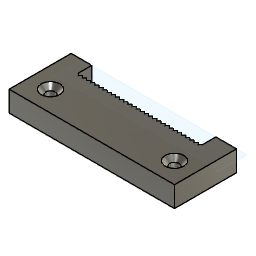
wall holder (Autodesk Fusion 360 design; units mm, degrees)
Autodesk Fusion 360 part; units mm, degrees
note: some values were not read from the file. Chosen so that the rebuilt part matches the saved one: which face or edge a step refers to.
sketch "Skizze1" plane through (0, 0, 0) normal (0, 0, 1) x (1, 0, 0)
  line L0 (0, 0) -> (80, 0)
  line L1 (80, 0) -> (80, -25)
  line L2 (80, -25) -> (0, -25)
  line L3 (0, -25) -> (0, 0)
  line L4 (40, -15) -> (40, -14)
  line L5 (40, -14) -> (39, -15)
  line L6 (38, -14) -> (39, -15)
  line L7 (38, -14) -> (37, -15)
  line L8 (37, -15) -> (36, -14)
  line L9 (36, -14) -> (35, -15)
  line L10 (35, -15) -> (34, -14)
  line L11 (34, -14) -> (33, -15)
  line L12 (33, -15) -> (32, -14)
  line L13 (32, -14) -> (31, -15)
  line L14 (31, -15) -> (30, -14)
  line L15 (30, -14) -> (29, -15)
  line L16 (29, -15) -> (28, -14)
  line L17 (28, -14) -> (27, -15)
  line L18 (27, -15) -> (26, -14)
  line L19 (26, -14) -> (25, -15)
  line L20 (25, -15) -> (24, -14)
  line L21 (24, -14) -> (23, -15)
  line L22 (23, -15) -> (22, -14)
  line L23 (22, -14) -> (21, -15)
  line L24 (21, -15) -> (20, -14)
  line L25 (20, -14) -> (19, -15)
  line L26 (19, -15) -> (18, -14)
  line L27 (18, -14) -> (17, -15)
  line L28 (17, -15) -> (16, -14)
  line L29 (16, -14) -> (15, -15)
  line L30 (15, -15) -> (14, -14)
  line L31 (14, -14) -> (13, -15)
  line L32 (13, -15) -> (12, -14)
  line L33 (12, -14) -> (11, -15)
  line L34 (11, -15) -> (10, -14)
  line L35 (10, -14) -> (9, -15)
  line L36 (9, -15) -> (8, -14)
  line L37 (8, -14) -> (7, -15)
  line L38 (7, -15) -> (6, -14)
  line L39 (6, -14) -> (5, -15)
  line L40 (5, -15) -> (4, -14)
  line L41 (4, -14) -> (3, -15)
  line L42 (3, -15) -> (2, -14)
  line L43 (2, -14) -> (1, -15)
  line L44 (40, -14) -> (41, -15)
  line L45 (41, -15) -> (42, -14)
  line L46 (42, -14) -> (43, -15)
  line L47 (43, -15) -> (44, -14)
  line L48 (44, -14) -> (45, -15)
  line L49 (45, -15) -> (46, -14)
  line L50 (46, -14) -> (47, -15)
  line L51 (47, -15) -> (48, -14)
  line L52 (48, -14) -> (49, -15)
  line L53 (49, -15) -> (50, -14)
  line L54 (50, -14) -> (51, -15)
  line L55 (51, -15) -> (52, -14)
  line L56 (52, -14) -> (53, -15)
  line L57 (53, -15) -> (54, -14)
  line L58 (54, -14) -> (55, -15)
  line L59 (55, -15) -> (56, -14)
  line L60 (56, -14) -> (57, -15)
  line L61 (57, -15) -> (58, -14)
  line L62 (58, -14) -> (59, -15)
  line L63 (59, -15) -> (60, -14)
  line L64 (60, -14) -> (61, -15)
  line L65 (61, -15) -> (62, -14)
  line L66 (62, -14) -> (63, -15)
  line L67 (63, -15) -> (64, -14)
  line L68 (64, -14) -> (65, -15)
  line L69 (65, -15) -> (66, -14)
  line L70 (66, -14) -> (67, -15)
  line L71 (67, -15) -> (68, -14)
  line L72 (68, -14) -> (69, -15)
  line L73 (69, -15) -> (70, -14)
  line L74 (70, -14) -> (71, -15)
  line L75 (71, -15) -> (72, -14)
  line L76 (72, -14) -> (73, -15)
  line L77 (73, -15) -> (74, -14)
  line L78 (74, -14) -> (75, -15)
  line L79 (75, -15) -> (76, -14)
  line L80 (76, -14) -> (77, -15)
  line L81 (77, -15) -> (78, -14)
  line L82 (78, -14) -> (79, -15)
  line L83 (1, -15) -> (0, -15)
  line L84 (79, -15) -> (80, -15)
  constraint horizontal L0
  constraint vertical L1
  constraint horizontal L2
  constraint vertical L3
  constraint coincident L0.start L3.end
  constraint perpendicular L6 L7
  constraint perpendicular L7 L8
  constraint perpendicular L8 L9
  constraint perpendicular L9 L10
  constraint perpendicular L10 L11
  constraint perpendicular L11 L12
  constraint perpendicular L12 L13
  constraint perpendicular L13 L14
  constraint perpendicular L14 L15
  constraint perpendicular L15 L16
  constraint perpendicular L16 L17
  constraint perpendicular L17 L18
  constraint perpendicular L18 L19
  constraint perpendicular L19 L20
  constraint perpendicular L20 L21
  constraint perpendicular L21 L22
  constraint perpendicular L22 L23
  constraint perpendicular L23 L24
  constraint perpendicular L24 L25
  constraint perpendicular L25 L26
  constraint perpendicular L26 L27
  constraint perpendicular L27 L28
  constraint perpendicular L28 L29
  constraint perpendicular L29 L30
  constraint perpendicular L30 L31
  constraint perpendicular L31 L32
  constraint perpendicular L32 L33
  constraint perpendicular L33 L34
  constraint perpendicular L34 L35
  constraint perpendicular L35 L36
  constraint perpendicular L36 L37
  constraint perpendicular L37 L38
  constraint perpendicular L38 L39
  constraint perpendicular L39 L40
  constraint perpendicular L40 L41
  constraint perpendicular L41 L42
  constraint perpendicular L42 L43
  constraint perpendicular L5 L44
  constraint perpendicular L44 L45
  constraint perpendicular L45 L46
  constraint perpendicular L46 L47
  constraint perpendicular L47 L48
  constraint perpendicular L48 L49
  constraint perpendicular L49 L50
  constraint perpendicular L50 L51
  constraint perpendicular L49 L52
  constraint perpendicular L52 L53
  constraint perpendicular L53 L54
  constraint perpendicular L54 L55
  constraint perpendicular L55 L56
  constraint perpendicular L56 L57
  constraint perpendicular L57 L58
  constraint perpendicular L58 L59
  constraint perpendicular L57 L60
  constraint perpendicular L60 L61
  constraint perpendicular L61 L62
  constraint perpendicular L62 L63
  constraint perpendicular L61 L64
  constraint perpendicular L64 L65
  constraint perpendicular L65 L66
  constraint perpendicular L66 L67
  constraint perpendicular L67 L68
  constraint perpendicular L68 L69
  constraint perpendicular L69 L70
  constraint perpendicular L70 L71
  constraint perpendicular L69 L72
  constraint perpendicular L72 L73
  constraint perpendicular L73 L74
  constraint perpendicular L74 L75
  constraint perpendicular L75 L76
  constraint perpendicular L76 L77
  constraint perpendicular L75 L78
  constraint perpendicular L78 L79
  constraint perpendicular L73 L80
  constraint perpendicular L80 L81
  constraint perpendicular L73 L82
  constraint coincident L3 L83.end
  constraint perpendicular L3 L83
  constraint coincident L1 L84.end
  constraint perpendicular L1 L84
extrude "Extrusion1" add sketch "Skizze1" along normal blind 10 draft 10 contours L1 L2 L3 L5 L6 L7 L8 L9 L10 L11 L12 L13 L14 L15 L16 L17 L18 L19 L20 L21 L22 L23 L24 L25 L26 L27 L28 L29 L30 L31 L32 L33 L34 L35 L36 L37 L38 L39 L40 L41 L42 L43 L44 L45 L46 L47 L48 L49 L50 L51 L52 L53 L54 L55 L56 L57 L58 L59 L60 L61 L62 L63 L64 L65 L66 L67 L68 L69 L70 L71 L72 L73 L74 L75 L76 L77 L78 L79 L80 L81 L82 L83 L84
sketch "Skizze2" plane through (0, 0, 0) normal (0, 0, 1) x (1, 0, 0)
  line L0 (0, -15) -> (0, 0)
  line L1 (0, 0) -> (80, 0)
  line L2 (80, 0) -> (80, -15)
  line L3 (80, -15) -> (0, -15)
  constraint coincident L0.end L1.start
  constraint vertical L0
  constraint perpendicular L0 L1
  constraint perpendicular L1 L2
  constraint perpendicular L0 L3
sketch "Skizze3" plane through (0, 0, 0) normal (0, 0, 1) x (1, 0, 0)
  line L0 (0, 0) -> (-15.5, 0)
  line L1 (-15.5, 0) -> (-15.5, -29)
  line L2 (-15.5, -29) -> (0, -29)
  line L3 (0, -29) -> (0, 0)
  constraint horizontal L0
  constraint vertical L1
  constraint horizontal L2
  constraint vertical L3
  constraint coincident L0.start L3.end
extrude "Extrusion3" cut sketch "Skizze3" along normal blind 11.5
sketch "Skizze4" plane through (0, 0, 0) normal (0, 0, 1) x (1, 0, 0)
  line L0 (80, 0) -> (90, 0)
  line L1 (90, 0) -> (90, -35)
  line L2 (90, -35) -> (80, -35)
  line L3 (80, -35) -> (80, 0)
  constraint horizontal L0
  constraint vertical L1
  constraint horizontal L2
  constraint vertical L3
extrude "Extrusion4" cut sketch "Skizze4" along normal blind 10
sketch "Skizze5" plane through (0, 0, 0) normal (0, 0, 1) x (1, 0, 0)
  line L0 (0, -25) -> (92, -25)
  line L1 (92, -25) -> (92, -42)
  line L2 (92, -42) -> (0, -42)
  line L3 (0, -42) -> (0, -25)
  constraint horizontal L0
  constraint vertical L1
  constraint horizontal L2
  constraint vertical L3
extrude "Extrusion5" cut sketch "Skizze5" along normal blind 13
sketch "Skizze6" plane through (0, 0, 5) normal (0, 0, 1) x (-1, 0, 0)
  line L0 (0, 14.1184) -> (-0.6348, 14.1184)
  line L1 (-0.6348, 14.1184) -> (-2, 12.7532)
  line L2 (-2, 12.7532) -> (-3, 13.7532)
  line L3 (-3, 13.7532) -> (-4, 12.7532)
  line L4 (-4, 12.7532) -> (-5, 13.7532)
  line L5 (-5, 13.7532) -> (-6, 12.7532)
  line L6 (-6, 12.7532) -> (-7, 13.7532)
  line L7 (-7, 13.7532) -> (-8, 12.7532)
  line L8 (-8, 12.7532) -> (-9, 13.7532)
  line L9 (-9, 13.7532) -> (-10, 12.7532)
  line L10 (-10, 12.7532) -> (-11, 13.7532)
  line L11 (-11, 13.7532) -> (-12, 12.7532)
  line L12 (-12, 12.7532) -> (-13, 13.7532)
  line L13 (-13, 13.7532) -> (-14, 12.7532)
  line L14 (-14, 12.7532) -> (-15, 13.7532)
  line L15 (-15, 13.7532) -> (-16, 12.7532)
  line L16 (-16, 12.7532) -> (-17, 13.7532)
  line L17 (-17, 13.7532) -> (-18, 12.7532)
  line L18 (-18, 12.7532) -> (-19, 13.7532)
  line L19 (-19, 13.7532) -> (-20, 12.7532)
  line L20 (-20, 12.7532) -> (-21, 13.7532)
  line L21 (-21, 13.7532) -> (-22, 12.7532)
  line L22 (-22, 12.7532) -> (-23, 13.7532)
  line L23 (-23, 13.7532) -> (-24, 12.7532)
  line L24 (-24, 12.7532) -> (-25, 13.7532)
  line L25 (-25, 13.7532) -> (-26, 12.7532)
  line L26 (-26, 12.7532) -> (-27, 13.7532)
  line L27 (-27, 13.7532) -> (-28, 12.7532)
  line L28 (-28, 12.7532) -> (-29, 13.7532)
  line L29 (-29, 13.7532) -> (-30, 12.7532)
  line L30 (-30, 12.7532) -> (-31, 13.7532)
  line L31 (-31, 13.7532) -> (-32, 12.7532)
  line L32 (-32, 12.7532) -> (-33, 13.7532)
  line L33 (-33, 13.7532) -> (-34, 12.7532)
  line L34 (-34, 12.7532) -> (-35, 13.7532)
  line L35 (-35, 13.7532) -> (-36, 12.7532)
  line L36 (-36, 12.7532) -> (-37, 13.7532)
  line L37 (-37, 13.7532) -> (-38, 12.7532)
  line L38 (-38, 12.7532) -> (-39, 13.7532)
  line L39 (-39, 13.7532) -> (-40, 12.7532)
  line L40 (-40, 12.7532) -> (-41, 13.7532)
  line L41 (-41, 13.7532) -> (-42, 12.7532)
  line L42 (-42, 12.7532) -> (-43, 13.7532)
  line L43 (-43, 13.7532) -> (-44, 12.7532)
  line L44 (-44, 12.7532) -> (-45, 13.7532)
  line L45 (-45, 13.7532) -> (-46, 12.7532)
  line L46 (-46, 12.7532) -> (-47, 13.7532)
  line L47 (-47, 13.7532) -> (-48, 12.7532)
  line L48 (-48, 12.7532) -> (-49, 13.7532)
  line L49 (-49, 13.7532) -> (-50, 12.7532)
  line L50 (-50, 12.7532) -> (-51, 13.7532)
  line L51 (-51, 13.7532) -> (-52, 12.7532)
  line L52 (-52, 12.7532) -> (-53, 13.7532)
  line L53 (-53, 13.7532) -> (-54, 12.7532)
  line L54 (-54, 12.7532) -> (-55, 13.7532)
  line L55 (-55, 13.7532) -> (-56, 12.7532)
  line L56 (-56, 12.7532) -> (-57, 13.7532)
  line L57 (-57, 13.7532) -> (-58, 12.7532)
  line L58 (-58, 12.7532) -> (-59, 13.7532)
  line L59 (-59, 13.7532) -> (-60, 12.7532)
  line L60 (-60, 12.7532) -> (-61, 13.7532)
  line L61 (-61, 13.7532) -> (-62, 12.7532)
  line L62 (-62, 12.7532) -> (-63, 13.7532)
  line L63 (-63, 13.7532) -> (-64, 12.7532)
  line L64 (-64, 12.7532) -> (-65, 13.7532)
  line L65 (-65, 13.7532) -> (-66, 12.7532)
  line L66 (-66, 12.7532) -> (-67, 13.7532)
  line L67 (-67, 13.7532) -> (-68, 12.7532)
  line L68 (-68, 12.7532) -> (-69, 13.7532)
  line L69 (-69, 13.7532) -> (-70, 12.7532)
  line L70 (-70, 12.7532) -> (-71, 13.7532)
  line L71 (-71, 13.7532) -> (-72, 12.7532)
  line L72 (-72, 12.7532) -> (-73, 13.7532)
  line L73 (-73, 13.7532) -> (-74, 12.7532)
  line L74 (-74, 12.7532) -> (-75, 13.7532)
  line L75 (-75, 13.7532) -> (-76, 12.7532)
  line L76 (-76, 12.7532) -> (-77, 13.7532)
  line L77 (-77, 13.7532) -> (-78, 12.7532)
  line L78 (-78, 12.7532) -> (-79.3652, 14.1184)
  line L79 (-79.3652, 14.1184) -> (-80, 14.1184)
  line L80 (-80, 14.1184) -> (-80, 0)
  line L81 (-80, 0) -> (0, 0)
  line L82 (0, 0) -> (0, 14.1184)
extrude "Extrusion6" add 1 faces at (53.3333, -25, 6.6667) along direction (0, -1, 0) blind 10
sketch "Skizze7" plane through (0, 0, 0) normal (0, 0, 1) x (1, 0, 0)
  line L0 (0, -15) -> (10, -15)
  line L1 (10, -15) -> (10, -5)
  line L2 (10, -5) -> (0, -5)
  line L3 (0, -5) -> (0, -15)
  line L4 (80, -15) -> (70, -15)
  line L5 (70, -15) -> (70, -5)
  line L6 (70, -5) -> (80, -5)
  line L7 (80, -5) -> (80, -15)
  constraint horizontal L0
  constraint vertical L1
  constraint horizontal L2
  constraint vertical L3
  constraint horizontal L4
  constraint vertical L5
  constraint horizontal L6
  constraint vertical L7
extrude "Extrusion7" add sketch "Skizze7" along normal blind 10
sketch "Skizze8" plane through (0, 0, 10) normal (0, 0, 1) x (-1, 0, 0)
  line L0 (0, 5) -> (0, 35)
  line L1 (0, 35) -> (-80, 35)
  line L2 (-80, 35) -> (-80, 5)
  line L3 (-80, 5) -> (-70, 5)
  line L4 (-70, 5) -> (-70, 11.5064)
  line L5 (-70, 11.5064) -> (-69, 12.5064)
  line L6 (-69, 12.5064) -> (-68, 11.5064)
  line L7 (-68, 11.5064) -> (-67, 12.5064)
  line L8 (-67, 12.5064) -> (-66, 11.5064)
  line L9 (-66, 11.5064) -> (-65, 12.5064)
  line L10 (-65, 12.5064) -> (-64, 11.5064)
  line L11 (-64, 11.5064) -> (-63, 12.5064)
  line L12 (-63, 12.5064) -> (-62, 11.5064)
  line L13 (-62, 11.5064) -> (-61, 12.5064)
  line L14 (-61, 12.5064) -> (-60, 11.5064)
  line L15 (-60, 11.5064) -> (-59, 12.5064)
  line L16 (-59, 12.5064) -> (-58, 11.5064)
  line L17 (-58, 11.5064) -> (-57, 12.5064)
  line L18 (-57, 12.5064) -> (-56, 11.5064)
  line L19 (-56, 11.5064) -> (-55, 12.5064)
  line L20 (-55, 12.5064) -> (-54, 11.5064)
  line L21 (-54, 11.5064) -> (-53, 12.5064)
  line L22 (-53, 12.5064) -> (-52, 11.5064)
  line L23 (-52, 11.5064) -> (-51, 12.5064)
  line L24 (-51, 12.5064) -> (-50, 11.5064)
  line L25 (-50, 11.5064) -> (-49, 12.5064)
  line L26 (-49, 12.5064) -> (-48, 11.5064)
  line L27 (-48, 11.5064) -> (-47, 12.5064)
  line L28 (-47, 12.5064) -> (-46, 11.5064)
  line L29 (-46, 11.5064) -> (-45, 12.5064)
  line L30 (-45, 12.5064) -> (-44, 11.5064)
  line L31 (-44, 11.5064) -> (-43, 12.5064)
  line L32 (-43, 12.5064) -> (-42, 11.5064)
  line L33 (-42, 11.5064) -> (-41, 12.5064)
  line L34 (-41, 12.5064) -> (-40, 11.5064)
  line L35 (-40, 11.5064) -> (-39, 12.5064)
  line L36 (-39, 12.5064) -> (-38, 11.5064)
  line L37 (-38, 11.5064) -> (-37, 12.5064)
  line L38 (-37, 12.5064) -> (-36, 11.5064)
  line L39 (-36, 11.5064) -> (-35, 12.5064)
  line L40 (-35, 12.5064) -> (-34, 11.5064)
  line L41 (-34, 11.5064) -> (-33, 12.5064)
  line L42 (-33, 12.5064) -> (-32, 11.5064)
  line L43 (-32, 11.5064) -> (-31, 12.5064)
  line L44 (-31, 12.5064) -> (-30, 11.5064)
  line L45 (-30, 11.5064) -> (-29, 12.5064)
  line L46 (-29, 12.5064) -> (-28, 11.5064)
  line L47 (-28, 11.5064) -> (-27, 12.5064)
  line L48 (-27, 12.5064) -> (-26, 11.5064)
  line L49 (-26, 11.5064) -> (-25, 12.5064)
  line L50 (-25, 12.5064) -> (-24, 11.5064)
  line L51 (-24, 11.5064) -> (-23, 12.5064)
  line L52 (-23, 12.5064) -> (-22, 11.5064)
  line L53 (-22, 11.5064) -> (-21, 12.5064)
  line L54 (-21, 12.5064) -> (-20, 11.5064)
  line L55 (-20, 11.5064) -> (-19, 12.5064)
  line L56 (-19, 12.5064) -> (-18, 11.5064)
  line L57 (-18, 11.5064) -> (-17, 12.5064)
  line L58 (-17, 12.5064) -> (-16, 11.5064)
  line L59 (-16, 11.5064) -> (-15, 12.5064)
  line L60 (-15, 12.5064) -> (-14, 11.5064)
  line L61 (-14, 11.5064) -> (-13, 12.5064)
  line L62 (-13, 12.5064) -> (-12, 11.5064)
  line L63 (-12, 11.5064) -> (-11, 12.5064)
  line L64 (-11, 12.5064) -> (-10, 11.5064)
  line L65 (-10, 11.5064) -> (-10, 5)
  line L66 (-10, 5) -> (0, 5)
  line L67 (-80, 35) -> (-70, 25)
  line L68 (0, 35) -> (-10, 25)
  constraint coincident L1.end L2.start
  constraint coincident L0.end L1.start
hole "Bohrung1" at (70, -25, 10) direction (0, 0, -1) diameter 4.5 depth 20 tip angle 180 countersink diameter 9 countersink angle 90
sketch "Skizze9" plane through (0, 0, 10) normal (0, 0, 1) x (-1, 0, 0)
  circle A0 centre (-70, 25) radius 4.5
  line L0 (0, 5) -> (0, 35)
  line L1 (0, 35) -> (-80, 35)
  line L2 (-80, 35) -> (-80, 5)
  line L3 (-80, 5) -> (-70, 5)
  line L4 (-70, 5) -> (-70, 11.5064)
  line L5 (-70, 11.5064) -> (-69, 12.5064)
  line L6 (-69, 12.5064) -> (-68, 11.5064)
  line L7 (-68, 11.5064) -> (-67, 12.5064)
  line L8 (-67, 12.5064) -> (-66, 11.5064)
  line L9 (-66, 11.5064) -> (-65, 12.5064)
  line L10 (-65, 12.5064) -> (-64, 11.5064)
  line L11 (-64, 11.5064) -> (-63, 12.5064)
  line L12 (-63, 12.5064) -> (-62, 11.5064)
  line L13 (-62, 11.5064) -> (-61, 12.5064)
  line L14 (-61, 12.5064) -> (-60, 11.5064)
  line L15 (-60, 11.5064) -> (-59, 12.5064)
  line L16 (-59, 12.5064) -> (-58, 11.5064)
  line L17 (-58, 11.5064) -> (-57, 12.5064)
  line L18 (-57, 12.5064) -> (-56, 11.5064)
  line L19 (-56, 11.5064) -> (-55, 12.5064)
  line L20 (-55, 12.5064) -> (-54, 11.5064)
  line L21 (-54, 11.5064) -> (-53, 12.5064)
  line L22 (-53, 12.5064) -> (-52, 11.5064)
  line L23 (-52, 11.5064) -> (-51, 12.5064)
  line L24 (-51, 12.5064) -> (-50, 11.5064)
  line L25 (-50, 11.5064) -> (-49, 12.5064)
  line L26 (-49, 12.5064) -> (-48, 11.5064)
  line L27 (-48, 11.5064) -> (-47, 12.5064)
  line L28 (-47, 12.5064) -> (-46, 11.5064)
  line L29 (-46, 11.5064) -> (-45, 12.5064)
  line L30 (-45, 12.5064) -> (-44, 11.5064)
  line L31 (-44, 11.5064) -> (-43, 12.5064)
  line L32 (-43, 12.5064) -> (-42, 11.5064)
  line L33 (-42, 11.5064) -> (-41, 12.5064)
  line L34 (-41, 12.5064) -> (-40, 11.5064)
  line L35 (-40, 11.5064) -> (-39, 12.5064)
  line L36 (-39, 12.5064) -> (-38, 11.5064)
  line L37 (-38, 11.5064) -> (-37, 12.5064)
  line L38 (-37, 12.5064) -> (-36, 11.5064)
  line L39 (-36, 11.5064) -> (-35, 12.5064)
  line L40 (-35, 12.5064) -> (-34, 11.5064)
  line L41 (-34, 11.5064) -> (-33, 12.5064)
  line L42 (-33, 12.5064) -> (-32, 11.5064)
  line L43 (-32, 11.5064) -> (-31, 12.5064)
  line L44 (-31, 12.5064) -> (-30, 11.5064)
  line L45 (-30, 11.5064) -> (-29, 12.5064)
  line L46 (-29, 12.5064) -> (-28, 11.5064)
  line L47 (-28, 11.5064) -> (-27, 12.5064)
  line L48 (-27, 12.5064) -> (-26, 11.5064)
  line L49 (-26, 11.5064) -> (-25, 12.5064)
  line L50 (-25, 12.5064) -> (-24, 11.5064)
  line L51 (-24, 11.5064) -> (-23, 12.5064)
  line L52 (-23, 12.5064) -> (-22, 11.5064)
  line L53 (-22, 11.5064) -> (-21, 12.5064)
  line L54 (-21, 12.5064) -> (-20, 11.5064)
  line L55 (-20, 11.5064) -> (-19, 12.5064)
  line L56 (-19, 12.5064) -> (-18, 11.5064)
  line L57 (-18, 11.5064) -> (-17, 12.5064)
  line L58 (-17, 12.5064) -> (-16, 11.5064)
  line L59 (-16, 11.5064) -> (-15, 12.5064)
  line L60 (-15, 12.5064) -> (-14, 11.5064)
  line L61 (-14, 11.5064) -> (-13, 12.5064)
  line L62 (-13, 12.5064) -> (-12, 11.5064)
  line L63 (-12, 11.5064) -> (-11, 12.5064)
  line L64 (-11, 12.5064) -> (-10, 11.5064)
  line L65 (-10, 11.5064) -> (-10, 5)
  line L66 (-10, 5) -> (0, 5)
  line L67 (0, 35) -> (-10, 25)
  constraint coincident L0.end L1.start
hole "Bohrung2" at (10, -25, 10) direction (0, 0, -1) diameter 4.5 depth 20 tip angle 180 countersink diameter 9 countersink angle 90
